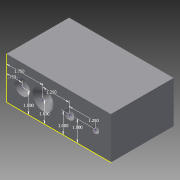
# Autodesk Inventor part: 7.2 Q4
Saved by Autodesk Inventor 2015 (Build 190159000, 159)
## iProperties
Created: 2018-02-12
Part Number: 7.2 Q4
Material: Generic
Document SubType Name: Modeling
Designer: Administrator
Density: 1 g/cm^3
Appearance: Default
Author: Administrator
Autodesk Inventor part; units mm, degrees
ref_plane "YZ Plane" through (0, 0, 0) normal (1, 0, 0) x (0, 1, 0)
ref_plane "XZ Plane" through (0, 0, 0) normal (0, 1, 0) x (-1, 0, 0)
ref_plane "XY Plane" through (0, 0, 0) normal (0, 0, 1) x (1, 0, 0)
sketch "Sketch1" plane through (0, 0, 0) normal (0, 0, 1) x (1, 0, 0)
  line L0 (0, 0) -> (127, 0)
  line L1 (127, 0) -> (127, 50.8)
  line L2 (127, 50.8) -> (0, 50.8)
  line L3 (0, 50.8) -> (0, 0)
  dimension "d0" = 50.8
  dimension "d1" = 127
  constraints: 8 end point, 2 parallel, 1 horizontal, 1 perpendicular
  measures "d0" distance of L2.end L0.start
  measures "d1" distance of L0.start L0.end
extrude "Extrusion1" add sketch "Sketch1" along normal blind 76.2
sketch "Sketch2" plane through (0, 0, 76.2) normal (0, 0, 1) x (1, 0, 0)
  line L0 (0, 0) -> (127, 0) projected
  line L1 (0, 50.8) -> (0, 0) projected
  point P0 (19.05, 25.4)
  point P1 (44.45, 25.4)
  point P2 (76.2, 25.4)
  point P3 (107.95, 25.4)
  dimension "d4" = 25.4
  dimension "d5" = 25.4
  dimension "d6" = 25.4
  dimension "d7" = 25.4
  dimension "d8" = 19.05
  dimension "d9" = 44.45
  dimension "d10" = 31.75
  dimension "d11" = 31.75
  measures "d4" distance from line of L0 point (19.05, 25.4)
  measures "d5" distance from line of L0 point (44.45, 25.4)
  measures "d6" distance from line of L0 point (76.2, 25.4)
  measures "d7" distance from line of L0 point (107.95, 25.4)
  measures "d8" distance from line of L1 point (19.05, 25.4)
  measures "d9" distance from line of L1 point (44.45, 25.4)
  measures "d10" distance of point (44.45, 25.4) point (76.2, 25.4)
  measures "d11" distance of point (107.95, 25.4) point (76.2, 25.4)
hole "Hole1" at (107.95, 25.4, 76.2) direction (0, 0, -1) diameter 6.35 depth 25.4 tip angle 118 counterbore diameter 9.525 counterbore depth 6.35
hole "Hole2" at (76.2, 25.4, 76.2) direction (0, 0, -1) diameter 12.7 end through all
hole "Hole3" at (44.45, 25.4, 76.2) direction (0, 0, -1) diameter 12.7 end through all countersink diameter 25.4 countersink angle 82
hole "Hole4" at (19.05, 25.4, 76.2) direction (0, 0, -1) diameter 12.7 depth 50.8 tip angle 118 counterbore diameter 19.05 counterbore depth 12.7
body "Solid1"
